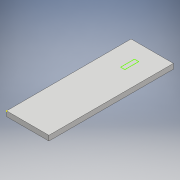
# Autodesk Inventor part: porte
Saved by Autodesk Inventor 2018 (Build 220112000, 112)
## iProperties
Created: 2018-11-21
Part Number: porte
Material: Generic
Document SubType Name: Modeling
Designer: Bienvenue
Density: 1 g/cm^3
Appearance: Default
Author: Bienvenue
Autodesk Inventor part; units mm, degrees
ref_plane "YZ Plane" through (0, 0, 0) normal (1, 0, 0) x (0, 1, 0)
ref_plane "XZ Plane" through (0, 0, 0) normal (0, 1, 0) x (-1, 0, 0)
ref_plane "XY Plane" through (0, 0, 0) normal (0, 0, 1) x (1, 0, 0)
sketch "Sketch1" plane through (0, 0, 0) normal (0, 0, 1) x (1, 0, 0)
  line L0 (0, 0) -> (170, 0)
  line L1 (170, 0) -> (170, 500)
  line L2 (170, 500) -> (0, 500)
  line L3 (0, 500) -> (0, 0)
  dimension "d0" = 170
  dimension "d1" = 500
  constraints: 8 end point, 2 parallel, 1 horizontal, 1 perpendicular
  measures "d0" distance of L1.end L2.end
  measures "d1" distance of L0.end L1.end
extrude "Extrusion1" add sketch "Sketch1" along normal blind 20
sketch "Sketch2" plane through (0, 0, 20) normal (0, 0, 1) x (1, 0, 0)
  line L0 (76.3289, 436.6253) -> (93.3645, 436.6253)
  line L1 (93.3645, 436.6253) -> (93.3645, 381.0355)
  line L2 (93.3645, 381.0355) -> (76.3289, 381.0355)
  line L3 (76.3289, 381.0355) -> (76.3289, 436.6253)
  point P0 (0, 0)
  constraints: 8 end point, 2 parallel, 1 horizontal, 1 perpendicular
body "Solid1"
